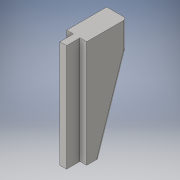
# Autodesk Inventor part: Right Leg, Side Partt
Saved by Autodesk Inventor 2016 (Build 200138000, 138)
## iProperties
Created: 2017-11-04
Part Number: Right Leg, Side Partt
Material: Generic
Document SubType Name: Modeling
Designer: mathaetaes
Density: 1 g/cm^3
Appearance: Default
Author: mathaetaes
Autodesk Inventor part; units mm, degrees
ref_plane "YZ Plane" through (0, 0, 0) normal (1, 0, 0) x (0, 1, 0)
ref_plane "XZ Plane" through (0, 0, 0) normal (0, 1, 0) x (-1, 0, 0)
ref_plane "XY Plane" through (0, 0, 0) normal (0, 0, 1) x (1, 0, 0)
sketch "Sketch1" plane through (0, 0, 0) normal (1, 0, 0) x (0, 1, 0)
  line L0 (45.2604, 28.0988) -> (45.2604, -22.7012)
  line L1 (45.2604, -22.7012) -> (19.8604, -22.7012)
  line L2 (19.8604, -22.7012) -> (-56.3396, 2.6988)
  line L3 (-56.3396, 2.6988) -> (-56.3396, 28.0988)
  line L4 (45.2604, 28.0988) -> (-56.3396, 28.0988)
  point P0 (0, 0)
  dimension "d0" = 50.8
  dimension "d1" = 25.4
  dimension "d2" = 76.2
  dimension "d3" = 25.4
  constraints: 10 end point, 1 horizontal, 1 parallel, 1 perpendicular, 1 vertical
  measures "d0" distance of L0.start L0.end
  measures "d1" distance of L2.end L3.end
  measures "d2" distance from line of L3 L1.end
  measures "d3" distance of L0.end L1.end
extrude "Extrusion1" add sketch "Sketch1" along normal blind 19.05
sketch "Sketch2" plane through (0, 45.2604, 28.0988) normal (0, 1, 0) x (1, 0, 0)
  line L0 (19.05, 50.8) -> (19.05, 0) projected
  line L1 (19.05, 0) -> (12.7, 0)
  line L2 (12.7, 0) -> (12.7, 12.7)
  line L3 (12.7, 12.7) -> (19.05, 12.7)
  line L4 (19.05, 12.7) -> (19.05, 0)
  line L5 (0, 0) -> (19.05, 0) projected
  line L6 (0, 0) -> (6.35, 0)
  line L7 (6.35, 0) -> (6.35, 12.7)
  line L8 (6.35, 12.7) -> (0, 12.7)
  line L9 (0, 12.7) -> (0, 0)
  point P0 (0, 28.0988)
  dimension "d6" = 6.35
  dimension "d7" = 12.7
  dimension "d8" = 6.35
  constraints: 16 end point, 4 parallel, 2 horizontal, 2 perpendicular, 1 point on line
  measures "d6" distance of L2.end L3.end
  measures "d7" distance of L1.end L2.end
  measures "d8" distance of L7.end L8.end
extrude "Extrusion2" cut sketch "Sketch2" against normal blind 101.6
fillet "Fillet1" radius 3.175 2 edges at (19.05, -18.2396, -10.0012) (19.05, 32.5604, -22.7012)
equation "\"d9\" = d3 + d2"
body "Solid1"
